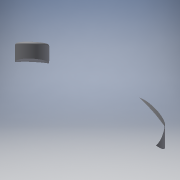
# Autodesk Inventor part: ojos
Saved by Autodesk Inventor 2016 (Build 200138000, 138)
## iProperties
Created: 2016-02-20
Part Number: ojos
Material: Genérico
Document SubType Name: Modeling
Designer: Usuario1
Density: 1 g/cm^3
Appearance: Valor por defecto
Author: Usuario1
Autodesk Inventor part; units mm, degrees
ref_plane "YZ Plane" through (0, 0, 0) normal (1, 0, 0) x (0, 1, 0)
ref_plane "XZ Plane" through (0, 0, 0) normal (0, 1, 0) x (-1, 0, 0)
ref_plane "XY Plane" through (0, 0, 0) normal (0, 0, 1) x (1, 0, 0)
sketch "Boceto1" plane through (0, 0, 0) normal (0, 0, 1) x (1, 0, 0)
  line L0 (-5.8393, 0) -> (0, 0)
  line L1 (-5.5036, 0.3) -> (0, 0.3)
  arc A0 (0, 5.3722) -> (-5.8393, 0) centre (0, -0.4875) ccw
  arc A1 (0, 5.0722) -> (-5.5036, 0.3) centre (0, -0.4875) ccw
  circle A2 centre (-2.7431, 2.581) radius 0.5709
  line L2 (0, 0) -> (0, 5.3722)
  line L3 (0, 5.3722) -> (0, 5.0722)
  line L4 (0, 0.3) -> (0, 0)
  constraints: 10 end point, 4 point on circle, 3 centre point, 2 point on line
extrude "Extrusión1" add sketch "Boceto1" along normal blind 8 contours A2
sketch "Boceto2" plane through (0, 0, 0) normal (0, 0, 1) x (1, 0, 0)
  line L0 (-5.8376, 0.0208) -> (0, 0.0208)
  line L1 (-5.5036, 0.3) -> (0, 0.3)
  arc A0 (0, 5.3722) -> (-5.8376, 0.0208) centre (0, -0.4875) ccw
  arc A1 (0, 5.0722) -> (-5.5036, 0.3) centre (0, -0.4875) ccw
  line L2 (0, 0.0208) -> (0, 5.3722)
  line L3 (0, 5.3722) -> (0, 5.0722)
  line L4 (0, 0.3) -> (0, 0.0208)
  line L5 (-15.8376, 0.0208) -> (-15.8376, 10.3501)
  line L6 (-15.8376, 10.3501) -> (0, 10.3501)
  arc A2 (0, 5.6222) -> (-6.0885, 0.0208) centre (0, -0.4875) ccw
  line L7 (-15.8376, 0.0208) -> (-6.0885, 0.0208)
  line L8 (0, 5.6222) -> (0, 10.3501)
  circle A3 centre (-2.7431, 2.581) radius 0.5709 projected
  point P0 (0, 0)
  point P1 (0, 0)
  dimension "d2" = 10
  dimension "d3" = 0.25
  constraints: 18 end point, 6 point on circle, 3 centre point, 2 perpendicular, 2 point on line, 1 horizontal
  measures "d2" distance of L0.start L5.start
  measures "d3" radial gap between concentric circles of A0 A2
revolve "Revolución1" cut sketch "Boceto2" angle 360 about axis through (0, 0.0208, 0) along (0, 1, 0) contours L1 A1 L2 | L5 L6 L8 A2 L7 | A3
fillet "Empalme2" radius 0.05 1 edges at (-3.3139, 2.5882, 4.1093)
mirror "Simetría2" about plane through (0, 0, 0) normal (1, 0, 0) of "Revolución1", "Extrusión1", "Empalme2"
